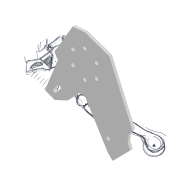
# Autodesk Inventor part: Knee
Saved by Autodesk Inventor 2020 (Build 240168000, 168)
## iProperties
Created: 2020-05-17
Part Number: Knee
Material: Generic
Document SubType Name: Sheet Metal
Designer: valer
Density: 1 g/cm^3
Sheet Metal Rule: Default
Appearance: Default
Author: valer
Autodesk Inventor part; units mm, degrees
ref_plane "YZ Plane" through (0, 0, 0) normal (1, 0, 0) x (0, 1, 0)
ref_plane "XZ Plane" through (0, 0, 0) normal (0, 1, 0) x (-1, 0, 0)
ref_plane "XY Plane" through (0, 0, 0) normal (0, 0, 1) x (1, 0, 0)
sketch "Base" plane through (0, 0, 0) normal (0, 0, 1) x (1, 0, 0)
  line L0 (0, 0) -> (-33.8953, -57.737)
  line L1 (22.7363, 2.3748) -> (0, 0)
  line L2 (68.6239, -13.5268) -> (22.7363, 2.3748)
  line L3 (-33.8953, -57.737) -> (-27.3376, -67.3369)
  line L4 (-27.3376, -67.3369) -> (-51.6074, -128.4874)
  line L5 (-51.6074, -128.4874) -> (-33.4288, -135.7023)
  line L6 (-27.3376, -67.3369) -> (12.1319, -101.41) construction
  line L7 (12.1319, -101.41) -> (22.7363, -100.8091)
  line L8 (12.1319, -101.41) -> (-9.1414, -124.4665)
  line L9 (-33.4288, -135.7023) -> (-9.1414, -124.4665)
  line L10 (22.7363, 2.3748) -> (68.6239, -13.5268)
  line L11 (68.6239, -13.5268) -> (112.0332, -112.3643)
  line L12 (22.7363, 2.3748) -> (22.7363, -100.8091) construction
  line L13 (22.7363, -100.8091) -> (65.9464, -171.1467)
  line L14 (112.0332, -112.3643) -> (104.5166, -122.601)
  line L15 (22.7363, -100.8091) -> (112.0332, -112.3643) construction
  circle A0 centre (22.7363, -49.2172) radius 38.1
  circle A1 centre (22.7363, -49.2172) radius 25.4 construction
  circle A2 centre (22.7363, -23.8172) radius 3.175
  line L16 (104.5166, -122.601) -> (102.8401, -135.301)
  line L17 (102.8401, -135.301) -> (107.7094, -147.0305)
  line L18 (65.9464, -171.1467) -> (74.9694, -180.0841)
  line L19 (107.7094, -147.0305) -> (74.9694, -180.0841)
  circle A3 centre (66.5926, -147.936) radius 25.4
  line L20 (-42.5181, -132.0949) -> (22.7363, -49.2172) construction
  line L21 (-33.0904, -120.1209) -> (-25.2339, -110.1427) construction
  line L22 (-35.5849, -118.1568) -> (-27.7285, -108.1786)
  line L23 (-22.7393, -112.1068) -> (-30.5958, -122.0851)
  arc A4 (-35.5849, -118.1568) -> (-30.5958, -122.0851) centre (-33.0904, -120.1209) ccw
  arc A5 (-22.7393, -112.1068) -> (-27.7285, -108.1786) centre (-25.2339, -110.1427) ccw
  circle A6 centre (0.7393, -36.5172) radius 3.175
  circle A7 centre (0.7393, -61.9172) radius 3.175
  circle A8 centre (22.7363, -74.6172) radius 3.175
  circle A9 centre (44.7334, -61.9172) radius 3.175
  circle A10 centre (44.7334, -36.5172) radius 3.175
  circle A11 centre (66.5926, -147.936) radius 3.175
  line L24 (0, -216.5758) -> (0, 38.8665)
  point P0 (-29.1621, -115.1318)
  dimension "d1" = 50.8
  dimension "d0" = 76.2
  dimension "d2" = 6.35
  dimension "d4" = 50.8
  dimension "d5" = 22.86
  dimension "d6" = 154.924
  dimension "d7" = 126.378
  dimension "d8" = 48.5647
  dimension "d9" = 66.9511
  dimension "d10" = 132.824
  dimension "d11" = 107.95
  dimension "d12" = 115.248
  dimension "d13" = 11.6259
  dimension "d14" = 65.7906
  dimension "d15" = 19.558
  dimension "d16" = 120
  dimension "d17" = 12.7
  dimension "d18" = 12.7
  dimension "d19" = 12.7
  dimension "d20" = 82.55
  dimension "d21" = 12.7
  dimension "d22" = 12.7
  dimension "d23" = 28.575
  dimension "d24" = 15.24
  dimension "d25" = 3.175
  dimension "d26" = 12.7
  dimension "d29" = 360
  dimension "d31" = 6.35
  dimension "d32" = 95.963
  dimension "d33" = 38.215
  dimension "d34" = 22.545
  dimension "d35" = 7.52
  dimension "d36" = 44.727
  dimension "d37" = 31.563
  dimension "d38" = 86.757
  dimension "d39" = 42.697
  dimension "d40" = 49.197
  dimension "d41" = 114.826
  measures "d0" diameter of A0
  measures "d2" diameter of A2
  measures "d4" diameter of A3
  measures "d5" distance of L1.start L1.end
  measures "d6" angle of L2 L1
  measures "d7" angle of L0 L1
  measures "d8" distance of L2.start L1.start
  measures "d9" distance of L1.end L3.start
  measures "d10" angle of L2 L11
  measures "d11" distance of L2.start L11.end
  measures "d12" angle of L0 L3
  measures "d13" distance of L3.start L3.end
  measures "d14" distance of L3.end L4.end
  measures "d15" distance of L4.end L5.end
  measures "d16" angle of L14 L11
  measures "d17" distance of L11.end L16.start
  measures "d18" vertical distance of L16.start L16.end
  measures "d19" distance of L16.end L19.start
  measures "d20" distance of L7.end L13.end
  measures "d21" distance of L13.end L18.end
  measures "d22" distance from line of L13 A3.centre
  measures "d23" distance from line of L19 A3.centre
  measures "d24" distance of L20.start L21.start
  measures "d25" radius of A4
  measures "d26" distance of L22.start L22.end
  measures "d31" diameter of A11
  measures "d32" angle of L24 L1
  measures "d33" angle of L24 L23
  measures "d34" angle of L17 L24
  measures "d35" angle of L16 L24
  measures "d36" angle of L19 L24
  measures "d37" angle of L13 L24
  measures "d38" angle of L7 L24
  measures "d39" angle of L8 L24
  measures "d40" angle of L6 L24
  measures "d41" angle of L9 L24
extrude "Plate1" add sketch "Base" along normal blind 5.08 contours L24 A0 L8 L9 L5 L4 L3 L0 | L1 L2 L11 L14 L16 L17 L19 L18 A3 L13 L7 L8 L24 A0 | L24 A6 A7 A0 | A0 L24 A7 A6 | A3 L18 L13 picked at (57.995, -152.133)
equation "\"d42\" = Thickness"
equation "\"BendRadius\" = Thickness"
equation "\"BendReliefWidth\" = Thickness"
equation "\"BendReliefDepth\" = 0.5 * Thickness"
equation "\"CornerReliefSize\" = 4 * Thickness"
equation "\"MinimumRemnant\" = 2 * Thickness"
equation "\"TransitionRadius\" = BendRadius"
equation "\"JacobiRadiusSize\" = BendRadius"
equation "\"GapSize\" = Thickness"
equation "\"Thickness\" = 5.08"
body "Solid1"
